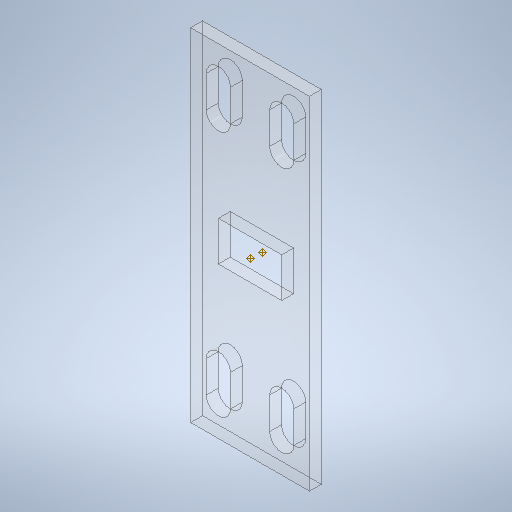
# Autodesk Inventor part: acrylic_temp_holder
Saved by Autodesk Inventor 2025 (Build 290162000, 162)
## iProperties
Created: 2024-04-25
Part Number: acrylic_temp_holder
Material: Polycarbonate, Clear
Document SubType Name: Modeling
Designer: warke
Density: 1.2 g/cm^3
Appearance: Polycarbonate - Clear
Author: warke
Autodesk Inventor part; units mm, degrees
ref_plane "YZ Plane" through (0, 0, 0) normal (1, 0, 0) x (0, 1, 0)
ref_plane "XZ Plane" through (0, 0, 0) normal (0, 1, 0) x (-1, 0, 0)
ref_plane "XY Plane" through (0, 0, 0) normal (0, 0, 1) x (1, 0, 0)
sketch "Sketch1" plane through (0, 0, 0) normal (0, 0, 1) x (1, 0, 0)
  circle A0 centre (4, 0) radius 1.0782 projected
  circle A1 centre (-4, 0) radius 1.0782 projected
  circle A2 centre (-4, -31.2) radius 1.0782 projected
  circle A3 centre (4, -31.2) radius 1.0782 projected
  line L0 (-7.5, -41.2) -> (7.5, -41.2) projected
  line L1 (7.5, -23.7) -> (7.5, -41.2) projected
  line L2 (7.5, -23.7) -> (2.5, -23.7) projected
  line L3 (2.5, -23.7) -> (2.5, -25.7) projected
  line L4 (2.5, -25.7) -> (-2.5, -25.7) projected
  line L5 (-2.5, -25.7) -> (-2.5, -23.7) projected
  line L6 (-2.5, -23.7) -> (-7.5, -23.7) projected
  line L7 (-7.5, -41.2) -> (-7.5, -23.7) projected
  circle A4 centre (4, -31.2) radius 1.0782 projected
  circle A5 centre (-4, -31.2) radius 1.0782 projected
  line L8 (7.5, 10) -> (-7.5, 10) projected
  line L9 (-7.5, -7.5) -> (-7.5, 10) projected
  line L10 (-7.5, -7.5) -> (-2.5, -7.5) projected
  line L11 (-2.5, -7.5) -> (-2.5, -5.5) projected
  line L12 (-2.5, -5.5) -> (2.5, -5.5) projected
  line L13 (2.5, -5.5) -> (2.5, -7.5) projected
  line L14 (2.5, -7.5) -> (7.5, -7.5) projected
  line L15 (7.5, 10) -> (7.5, -7.5) projected
  circle A6 centre (-4, 0) radius 1.0782 projected
  circle A7 centre (4, 0) radius 1.0782 projected
  line L16 (7.5, 10) -> (7.5, 6)
  line L17 (7.5, 6) -> (-7.5, 6)
  line L18 (5.524, 2) -> (5.524, -2)
  line L19 (2.476, -2) -> (2.476, 2)
  arc A8 (5.524, 2) -> (2.476, 2) centre (4, 2) ccw
  arc A9 (2.476, -2) -> (5.524, -2) centre (4, -2) ccw
  line L20 (-2.476, 2) -> (-2.476, -2)
  line L21 (-5.524, -2) -> (-5.524, 2)
  arc A10 (-2.476, 2) -> (-5.524, 2) centre (-4, 2) ccw
  arc A11 (-5.524, -2) -> (-2.476, -2) centre (-4, -2) ccw
  line L22 (5.524, 2) -> (5.524, -2)
  line L23 (2.476, -2) -> (2.476, 2)
  arc A12 (5.524, 2) -> (2.476, 2) centre (4, 2) ccw
  arc A13 (2.476, -2) -> (5.524, -2) centre (4, -2) ccw
  line L24 (5.524, -29.2) -> (5.524, -33.2)
  line L25 (2.476, -33.2) -> (2.476, -29.2)
  arc A14 (5.524, -29.2) -> (2.476, -29.2) centre (4, -29.2) ccw
  arc A15 (2.476, -33.2) -> (5.524, -33.2) centre (4, -33.2) ccw
  line L26 (-2.476, -29.2) -> (-2.476, -33.2)
  line L27 (-5.524, -33.2) -> (-5.524, -29.2)
  arc A16 (-2.476, -29.2) -> (-5.524, -29.2) centre (-4, -29.2) ccw
  arc A17 (-5.524, -33.2) -> (-2.476, -33.2) centre (-4, -33.2) ccw
  line L28 (7.5, -41.2) -> (7.5, -37.2)
  line L29 (7.5, -37.2) -> (-7.5, -37.2)
  line L30 (-7.5, 6) -> (-7.5, -37.2)
  line L31 (7.5, -37.2) -> (7.5, 6)
  line L32 (7.5, -7.5) -> (2.5, -7.5) projected
  line L33 (2.5, -7.5) -> (2.5, -5.5) projected
  line L34 (2.5, -5.5) -> (-2.5, -5.5) projected
  line L35 (-2.5, -5.5) -> (-2.5, -7.5) projected
  line L36 (-2.5, -7.5) -> (-7.5, -7.5) projected
  line L37 (-7.5, -12.5) -> (-7.5, -7.5) projected
  line L38 (5.5, -15) -> (-5.5, -15) projected
  line L39 (7.5, -7.5) -> (7.5, -12.5) projected
  line L40 (6.5, -16.2) -> (7.5, -18.7) projected
  line L41 (-7.5, -23.7) -> (-2.5, -23.7) projected
  line L42 (-2.5, -23.7) -> (-2.5, -25.7) projected
  line L43 (-2.5, -25.7) -> (2.5, -25.7) projected
  line L44 (2.5, -25.7) -> (2.5, -23.7) projected
  line L45 (2.5, -23.7) -> (7.5, -23.7) projected
  line L46 (7.5, -18.7) -> (7.5, -23.7) projected
  line L47 (-5.5, -16.2) -> (5.5, -16.2) projected
  line L48 (-7.5, -23.7) -> (-7.5, -18.7) projected
  line L49 (6.5, -15) -> (7.5, -12.5)
  line L50 (6.5, -16.2) -> (7.5, -18.7)
  line L51 (4, -13.1) -> (-4, -13.1)
  line L52 (-4, -13.1) -> (-4, -18.1)
  line L53 (-4, -18.1) -> (4, -18.1)
  line L54 (4, -18.1) -> (4, -13.1)
  line L55 (4, -13.1) -> (-4, -18.1) construction
  line L56 (-4, -13.1) -> (4, -18.1) construction
  line L57 (-1.5, -15) -> (1.5, -15)
  line L58 (1.5, -15) -> (1.5, -16.2)
  line L59 (1.5, -16.2) -> (-1.5, -16.2)
  line L60 (-1.5, -16.2) -> (-1.5, -15)
  line L61 (-1.5, -15) -> (1.5, -16.2) construction
  line L62 (1.5, -15) -> (-1.5, -16.2) construction
  line L63 (5.5, -12.5) -> (7.5, -12.5) projected
  line L64 (-7.5, -12.5) -> (-5.5, -12.5) projected
  line L65 (-5.5, -12.5) -> (-5.5, -15) projected
  line L66 (5.5, -15) -> (5.5, -12.5) projected
  line L67 (-5.5, -18.7) -> (-7.5, -18.7) projected
  line L68 (7.5, -18.7) -> (5.5, -18.7) projected
  line L69 (5.5, -18.7) -> (5.5, -16.2) projected
  line L70 (-5.5, -16.2) -> (-5.5, -18.7) projected
  point P0 (0, 0)
  point P1 (0, -15.6)
  point P2 (7.5, -7.5)
  point P3 (-7.5, -23.7)
  dimension "d0" = 4
  dimension "d5" = 4
  dimension "d6" = 8
  dimension "d7" = 5
  dimension "d10" = 3
  constraints: 60 end point, 20 point on circle, 15 tangent, 10 centre point, 5 perpendicular, 5 point on line, 4 midpoint, 4 parallel, 2 horizontal, 1 collinear
  measures "d0" distance of L8.start L16.end
  measures "d5" distance of L0.end L28.end
  measures "d6" distance of L53.end L52.end
  measures "d7" distance of L52.end L51.end
  measures "d10" distance of L58.end L59.end
extrude "Extrusion1" add sketch "Sketch1" along normal blind 1.5 contours L7 L6 L5 L4 L3 L2 L1 L29 | L30 L67 L70 L47 L52 L53 L54 L69 L68 L31 L2 L3 L4 L5 L6 | L30 L64 L65 L38 L52 L47 L70 L67 | L68 L69 L47 L54 L38 L66 L63 L31 | L30 L10 L11 L12 L13 L14 L31 L63 L66 L38 L54 L51 L52 L65 L64 | L9 L17 L15 L14 L13 L12 L11 L10
body "Solid1"
